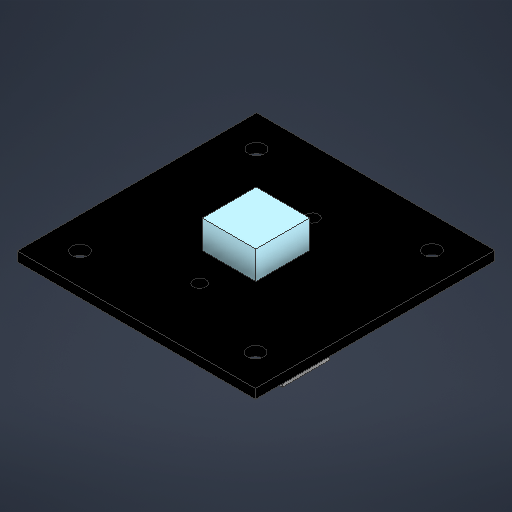
# Autodesk Inventor part: Camera
Saved by Autodesk Inventor 2025.1 (Build 291241000, 241)
## iProperties
Created: 2024-11-08
Part Number: Camera
Material: Generic
Document SubType Name: Modeling
Designer: jerem
Density: 1 g/cm^3
Appearance: Default
Author: jerem
Autodesk Inventor part; units mm, degrees
ref_plane "YZ Plane" through (0, 0, 0) normal (1, 0, 0) x (0, 1, 0)
ref_plane "XZ Plane" through (0, 0, 0) normal (0, 1, 0) x (-1, 0, 0)
ref_plane "XY Plane" through (0, 0, 0) normal (0, 0, 1) x (1, 0, 0)
sketch "Sketch1" plane through (0, 0, 0) normal (0, 1, 0) x (-1, 0, 0)
  line L0 (-19, -19.1) -> (19, -19.1)
  line L1 (19, -19.1) -> (19, 19.1)
  line L2 (19, 19.1) -> (-19, 19.1)
  line L3 (-19, 19.1) -> (-19, -19.1)
  line L4 (-19, -19.1) -> (19, 19.1) construction
  line L5 (19, -19.1) -> (-19, 19.1) construction
  line L6 (4.275, -4.2975) -> (-4.275, -4.2975)
  line L7 (-4.275, -4.2975) -> (-4.275, 4.2975)
  line L8 (-4.275, 4.2975) -> (4.275, 4.2975)
  line L9 (4.275, 4.2975) -> (4.275, -4.2975)
  line L10 (4.275, -4.2975) -> (-4.275, 4.2975) construction
  line L11 (-4.275, -4.2975) -> (4.275, 4.2975) construction
  circle A0 centre (14, 14.0737) radius 1.3
  circle A1 centre (0, 9) radius 1
  circle A2 centre (-14, 14.0737) radius 1.3
  circle A3 centre (0, -9) radius 1
  line L12 (0, 0) -> (0, 9) construction
  line L13 (0, -9) -> (0, 0) construction
  circle A4 centre (14, -14.0737) radius 1.3
  circle A5 centre (-14, -14.0737) radius 1.3
  line L14 (14, 14.0737) -> (14, -14.0737) construction
  line L15 (14, 14.0737) -> (-14, 14.0737) construction
  line L16 (-14, 14.0737) -> (-14, -14.0737) construction
  dimension "d0" = 38
  dimension "d1" = 38.2
  dimension "d2" = 8.55
  dimension "d3" = 2
  dimension "d4" = 2
  dimension "d5" = 9
  dimension "d6" = 9
  dimension "d7" = 2.6
  dimension "d8" = 2.6
  dimension "d9" = 2.6
  dimension "d10" = 2.6
  dimension "d11" = 28
  constraints: 35 end point, 6 centre point, 5 point on line, 4 midpoint, 4 parallel, 4 vertical, 3 horizontal, 2 perpendicular
  measures "d0" distance of L2.end L1.end
  measures "d1" distance of L0.end L1.end
  measures "d2" distance of L7.end L8.end
  measures "d3" diameter of A1
  measures "d4" diameter of A3
  measures "d5" distance of L12.start L13.start
  measures "d6" distance of L12.start L12.end
  measures "d7" diameter of A0
  measures "d8" diameter of A4
  measures "d9" diameter of A2
  measures "d10" diameter of A5
  measures "d11" distance of L14.start L15.end
extrude "Extrusion1" add sketch "Sketch1" along normal blind 1.5 contours L3 L2 L1 L0 | L6 L7 L8 L9
extrude "Extrusion2" add sketch "Sketch1" along normal blind 4.5 from surface at 1.5 contours L6 L7 L8 L9
sketch "Sketch2" plane through (0, 0, 0) normal (0, -1, 0) x (1, 0, 0)
  line L0 (15, 10.78) -> (11.5, 10.78)
  line L1 (11.5, 10.78) -> (11.5, 3.28)
  line L2 (11.5, 3.28) -> (15, 3.28)
  line L3 (15, 3.28) -> (15, 10.78)
  line L4 (-19, 19.1) -> (19, 19.1) projected
  line L5 (19, 19.1) -> (19, -19.1) projected
  line L6 (11.9, 3.68) -> (11.9, 10.38)
  line L7 (11.9, 10.38) -> (14.6, 10.38)
  line L8 (14.6, 10.38) -> (14.6, 3.68)
  line L9 (14.6, 3.68) -> (11.9, 3.68)
  point P0 (0, 0)
  dimension "d16" = 8.32
  dimension "d17" = 7.5
  dimension "d18" = 3.5
  dimension "d19" = 4
  dimension "d23" = 0.4
  constraints: 16 end point, 4 parallel, 2 perpendicular, 1 horizontal, 3 other
  measures "d16" distance between parallel lines of L4 L0
  measures "d17" distance of L0.end L1.end
  measures "d18" distance of L1.end L2.end
  measures "d19" distance between parallel lines of L5 L3
  measures "d23" distance between parallel lines of L1 L6
extrude "Extrusion3" add sketch "Sketch2" along normal blind 4.5
equation "\"d4\" = d3"
equation "\"d5\" = d6"
equation "\"d8\" = d7"
equation "\"d9\" = d7"
equation "\"d10\" = d7"
body "Solid1"
